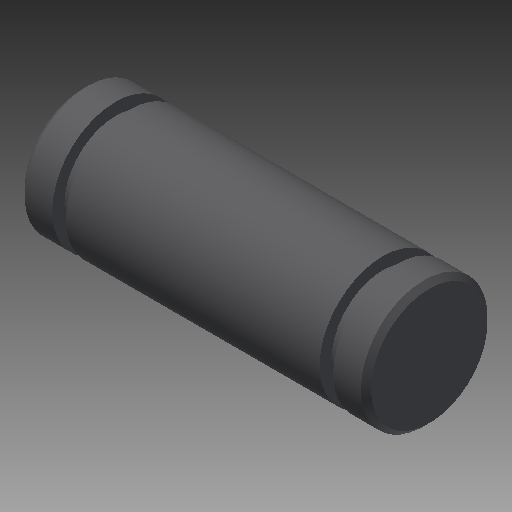
# Autodesk Inventor part: D-8383
Saved by Autodesk Inventor 2017 (Build 210142000, 142)
## iProperties
Category: PARTsolutions
Company: BIMBA
Created: 2016-10-01
Part Number: D-8383
Catalog Web Link: www.cadenas.de
Description: Piston Rod Clevis for Original Line Cylinders - Pin-
Vendor: BIMBA
Document SubType Name: Modeling
Designer: psAdmin
Manufacturer: BIMBA
Mass: 1.8256 g
Surface Area: 10.0418 cm^2
Volume: 1.8256 cm^3
Density: 1 g/cm^3
Material: Generic
Appearance: PSOLRGB-191-191-191
PSOL_IDENT_0: {$CADENAS_DATA\23d-libs\bimba\bimba\bimba_imperial\bimba_full_line\original_line_cylinders\accessori
PSOL_IDENT_1: es\piston_rod_clevis_pin.prj},199 {VTYP=3D},{NB=D-8383},{LINA=D-8383},{NN=Piston Rod Clevis for Orig
PSOL_IDENT_2: inal Line Cylinders - Pin},{DATE=22.09.2016 13:52:23},{GEOMDATE=03.04.2013 12:23:00},{VERSION=},{LIN
PSOL_IDENT_3: EID=40},{LINESUBID=-1},{WBVAR=}  {NB=D-8383},{LINA=D-8383},{KT=DUMMY},{PN=D-8383},{L=1.03100000},{L1=
PSOL_IDENT_4: 0.75500000},{L2=0.04050000},{L4=0.09800000},{D=0.37650000},{D1=0.30450000},{CH=0.01500000},{R=0.0025
PSOL_IDENT_5: 0000},{COLOR=0.75,0.75,0.75,0.00}
NN: Piston Rod Clevis for Original Line Cylinders - Pin
NB: D-8383
NBSYN: $PN.
LINA: D-8383
PN: D-8383
L: 1.03100000
L1: 0.75500000
L2: 0.04050000
L4: 0.09800000
D: 0.37650000
D1: 0.30450000
CH: 0.01500000
R: 0.00250000
SUPPLIER: BIMBA
ARTICLENO: D-8383
BOMINFO: D-8383
CREATOR: CADENAS GmbH
Title: D-8383
Author: Cadenas PARTsolutions
Autodesk Inventor part; units mm, degrees
sketch "Sketch_1" plane through (0, 0, 0) normal (0, 0, 1) x (1, 0, 0)
  line L0 (13.0937, 0) -> (-13.0937, 0)
  line L1 (-13.0937, 0) -> (-13.0937, 4.4005)
  line L2 (-13.0937, 4.4005) -> (-12.7127, 4.7816)
  line L3 (-12.7127, 4.7816) -> (-10.6172, 4.7816)
  line L4 (-10.6172, 4.7816) -> (-10.6172, 3.8672)
  line L5 (-10.6172, 3.8672) -> (-9.5885, 3.8672)
  line L6 (-9.5885, 3.8672) -> (-9.5885, 4.7816)
  line L7 (-9.5885, 4.7816) -> (9.5885, 4.7816)
  line L8 (9.5885, 4.7816) -> (9.5885, 3.8672)
  line L9 (9.5885, 3.8672) -> (10.6172, 3.8672)
  line L10 (10.6172, 3.8672) -> (10.6172, 4.7816)
  line L11 (10.6172, 4.7816) -> (12.7127, 4.7816)
  line L12 (12.7127, 4.7816) -> (13.0937, 4.4005)
  line L13 (13.0937, 4.4005) -> (13.0937, 0)
  line L14 (13.0937, 0) -> (-13.0937, 0)
  constraints: 30 end point
revolve "Revolution1" add sketch "Sketch_1" angle 360 about axis through (13.0937, 0, 0) along (1, 0, 0)
ref_plane "p1_XY" through (0, 0, 4.7816) normal (1, 0, 0) x (0, 0, -1)
ref_plane "p1_YZ" through (0, 0, 4.7816) normal (0, 0, -1) x (0, 1, 0)
ref_plane "p1_ZX" through (0, 0, 4.7816) normal (0, 1, 0) x (1, 0, 0)
ref_plane "p2_XY" through (0, 0, -4.7816) normal (1, 0, 0) x (0, 0, -1)
ref_plane "p2_YZ" through (0, 0, -4.7816) normal (0, 0, -1) x (0, 1, 0)
ref_plane "p2_ZX" through (0, 0, -4.7816) normal (0, 1, 0) x (1, 0, 0)
ref_plane "pin_XY" through (0, 0, 0) normal (1, 0, 0) x (0, 0, -1)
ref_plane "pin_YZ" through (0, 0, 0) normal (0, 0, -1) x (0, 1, 0)
ref_plane "pin_ZX" through (0, 0, 0) normal (0, 1, 0) x (1, 0, 0)
ref_plane "rr1_XY" through (10.1029, 0, 0) normal (1, 0, 0) x (0, 0, -1)
ref_plane "rr1_YZ" through (10.1029, 0, 0) normal (0, 0, -1) x (0, 1, 0)
ref_plane "rr1_ZX" through (10.1029, 0, 0) normal (0, 1, 0) x (1, 0, 0)
ref_plane "rr2_XY" through (-10.1029, 0, 0) normal (1, 0, 0) x (0, 0, -1)
ref_plane "rr2_YZ" through (-10.1029, 0, 0) normal (0, 0, -1) x (0, 1, 0)
ref_plane "rr2_ZX" through (-10.1029, 0, 0) normal (0, 1, 0) x (1, 0, 0)
ref_plane "w21_XY" through (13.0937, 0, 0) normal (0, 1, 0) x (1, 0, 0)
ref_plane "w21_YZ" through (13.0937, 0, 0) normal (1, 0, 0) x (0, 0, -1)
ref_plane "w21_ZX" through (13.0937, 0, 0) normal (0, 0, -1) x (0, 1, 0)
ref_plane "w22_XY" through (-13.0937, 0, 0) normal (0, 1, 0) x (1, 0, 0)
ref_plane "w22_YZ" through (-13.0937, 0, 0) normal (1, 0, 0) x (0, 0, -1)
ref_plane "w22_ZX" through (-13.0937, 0, 0) normal (0, 0, -1) x (0, 1, 0)
body "Solid1"
